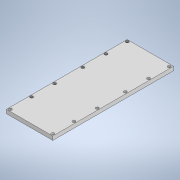
# Autodesk Inventor part: Floor_Final
Saved by Autodesk Inventor 2022 (Build 260153000, 153)
## iProperties
Created: 2023-01-11
Part Number: Floor_Final
Material: Generic
Document SubType Name: Modeling
Designer: s151859
Density: 1 g/cm^3
Appearance: Default
Author: s151859
Autodesk Inventor part; units mm, degrees
ref_plane "YZ Plane" through (0, 0, 0) normal (1, 0, 0) x (0, 1, 0)
ref_plane "XZ Plane" through (0, 0, 0) normal (0, 1, 0) x (-1, 0, 0)
ref_plane "XY Plane" through (0, 0, 0) normal (0, 0, 1) x (1, 0, 0)
sketch "Sketch1" plane through (0, 0, 0) normal (0, 1, 0) x (-1, 0, 0)
  line L0 (33.144, 98.7711) -> (-43.056, 98.7711)
  line L1 (-43.056, 98.7711) -> (-43.056, -99.9839)
  line L2 (-43.056, -99.9839) -> (33.144, -99.9839)
  line L3 (33.144, -99.9839) -> (33.144, 98.7711)
  point P0 (0, 0)
  dimension "d0" = 198.755
  dimension "d1" = 76.2
  constraints: 8 end point, 2 parallel, 1 horizontal, 1 perpendicular
  measures "d0" distance of L0.end L1.end
  measures "d1" distance of L0.start L0.end
extrude "Extrusion1" add sketch "Sketch1" along normal blind 6.35
sketch "Sketch2" plane through (0, 6.35, 0) normal (0, 1, 0) x (1, 0, 0)
  circle A0 centre (-29.969, 23.7839) radius 2.3813
  circle A1 centre (-29.969, -60.6711) radius 2.3813
  circle A2 centre (-29.969, -95.5961) radius 2.3813
  circle A3 centre (39.881, 61.8839) radius 2.3813
  circle A4 centre (39.881, 23.7839) radius 2.3813
  circle A5 centre (39.881, -60.6711) radius 2.3813
  circle A6 centre (39.881, 95.8575) radius 2.3813
  circle A7 centre (-29.969, 96.8089) radius 2.3813
  circle A8 centre (39.881, -95.5961) radius 2.3813
  circle A9 centre (-29.969, 61.8839) radius 2.3813
  line L0 (-33.144, 99.9839) -> (-33.144, -98.7711) projected
  line L1 (43.056, 99.9839) -> (-33.144, 99.9839) projected
  line L2 (43.056, -98.7711) -> (43.056, 99.9839) projected
  line L3 (-33.144, -98.7711) -> (43.056, -98.7711) projected
  circle A10 centre (-29.969, -22.5711) radius 2.3813
  circle A11 centre (39.881, -22.5711) radius 2.3813
  point P0 (0, 0)
  dimension "d4" = 3.175
  dimension "d5" = 3.175
  dimension "d6" = 3.175
  dimension "d7" = 3.175
  dimension "d8" = 3.175
  dimension "d9" = 3.175
  dimension "d10" = 3.175
  dimension "d11" = 3.175
  dimension "d12" = 3.175
  dimension "d13" = 3.175
  dimension "d14" = 3.175
  dimension "d15" = 3.175
  dimension "d16" = 3.175
  dimension "d17" = 38.1
  dimension "d18" = 76.2
  dimension "d19" = 38.1
  dimension "d20" = 38.1
  dimension "d21" = 38.1
  dimension "d22" = 76.2
  dimension "d23" = 76.2
  dimension "d24" = 3.175
  dimension "d25" = 76.2
  dimension "d26" = 3.175
  constraints: 12 centre point
  measures "d4" distance from line of L0 A7.centre
  measures "d5" distance from line of L1 A7.centre
  measures "d6" distance from line of L2 A6.centre
  measures "d7" distance from line of L2 A3.centre
  measures "d8" distance from line of L2 A4.centre
  measures "d9" distance from line of L2 A5.centre
  measures "d10" distance from line of L2 A8.centre
  measures "d11" distance from line of L3 A8.centre
  measures "d12" distance from line of L0 A2.centre
  measures "d13" distance from line of L3 A2.centre
  measures "d14" distance from line of L0 A1.centre
  measures "d15" distance from line of L0 A0.centre
  measures "d16" distance from line of L0 A9.centre
  measures "d17" distance from line of L1 A3.centre
  measures "d18" distance from line of L1 A4.centre
  measures "d19" distance from line of L3 A5.centre
  measures "d20" distance from line of L3 A1.centre
  measures "d21" distance from line of L1 A9.centre
  measures "d22" distance from line of L1 A0.centre
  measures "d23" distance from line of L3 A10.centre
  measures "d24" distance from line of L0 A10.centre
  measures "d25" distance from line of L3 A11.centre
  measures "d26" distance from line of L2 A11.centre
extrude "Extrusion2" cut sketch "Sketch2" against normal blind 11.1125 contours A0 | A1 | A2 | A3 | A4 | A5 | A6 | A7 | A8 | A9 | A10 | A11
body "Solid1"
